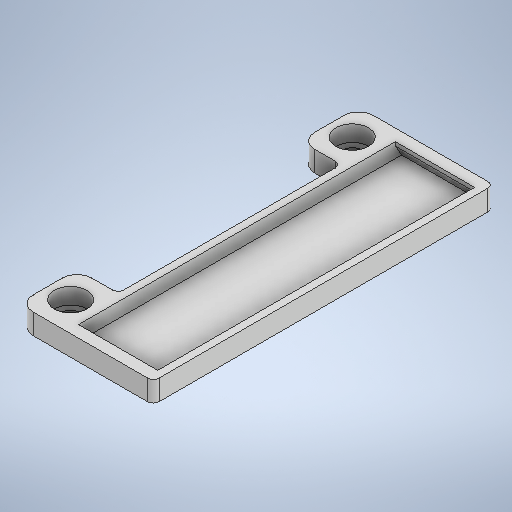
# Autodesk Inventor part: Bracket Clamp
Saved by Autodesk Inventor 2025 (Build 290162000, 162)
## iProperties
Created: 2025-03-11
Part Number: Bracket Clamp
Material: Generic
Document SubType Name: Modeling
Designer: Caleb Fangmeier
Density: 1 g/cm^3
Appearance: Default
Author: Caleb Fangmeier
Autodesk Inventor part; units mm, degrees
ref_plane "YZ Plane" through (0, 0, 0) normal (1, 0, 0) x (0, 1, 0)
ref_plane "XZ Plane" through (0, 0, 0) normal (0, 1, 0) x (-1, 0, 0)
ref_plane "XY Plane" through (0, 0, 0) normal (0, 0, 1) x (1, 0, 0)
sketch "Sketch1" plane through (0, 0, 0) normal (0, 1, 0) x (-1, 0, 0)
  line L0 (-16, 58) -> (16, 58)
  line L1 (16, 58) -> (16, -58)
  line L2 (16, -58) -> (-16, -58)
  line L3 (-16, -58) -> (-16, 58)
  line L4 (-16, 58) -> (16, -58) construction
  line L5 (16, 58) -> (-16, -58) construction
  point P0 (0, 0)
  dimension "d0" = 32
  dimension "d1" = 116
  constraints: 12 end point, 2 midpoint, 2 parallel, 1 horizontal, 1 perpendicular
  measures "d0" distance of L1.end L2.end
  measures "d1" distance of L0.end L1.end
extrude "Extrusion1" add sketch "Sketch1" along normal blind 7
sketch "Sketch3" plane through (16, 0, 58) normal (1, 0, 0) x (0, 0, -1)
  line L0 (0, 7) -> (116, 7) projected
  line L1 (4.75, 7) -> (1.8632, 2)
  line L2 (1.8632, 2) -> (114.1368, 2)
  line L3 (114.1368, 2) -> (111.25, 7)
  line L4 (0, 0) -> (0, 7) projected
  line L5 (116, 0) -> (116, 7) projected
  line L6 (4, 5.701) -> (4, 7)
  line L7 (116, 7) -> (0, 7) projected
  line L8 (112, 7) -> (112, 5.701)
  point P0 (58, 0)
  dimension "d4" = 60
  dimension "d6" = 60
  dimension "d7" = 5
  dimension "d8" = 106.5
  dimension "d9" = 116
  dimension "d10" = 4.75
  dimension "d17" = 4
  dimension "d18" = 4
  constraints: 10 end point, 6 point on line, 2 perpendicular, 1 horizontal
  measures "d4" angle of L2 L1
  measures "d6" angle of L2 L3
  measures "d7" distance between parallel lines of L0 L2
  measures "d8" distance of L1.start L3.end
  measures "d9" distance between parallel lines of L4 L5
  measures "d10" distance of L0.start L1.start
  measures "d17" distance between parallel lines of L4 L6
  measures "d18" distance between parallel lines of L8 L5
extrude "Extrusion2" cut sketch "Sketch3" against normal through all
sketch "Sketch4" plane through (0, 7, 0) normal (0, 1, 0) x (1, 0, 0)
  line L0 (-16, 58) -> (-16, -58) projected
  line L1 (-16, -58) -> (-13.5, -58)
  line L2 (-13.5, -58) -> (-13.5, 58)
  line L3 (-13.5, 58) -> (-16, 58)
  line L4 (-16, 58) -> (-16, -58)
  line L5 (16, -58) -> (16, 58) projected
  line L6 (16, -58) -> (13.5, -58)
  line L7 (13.5, -58) -> (13.5, 58)
  line L8 (13.5, 58) -> (16, 58)
  line L9 (16, 58) -> (16, -58)
  line L10 (16, 58) -> (-16, 58) projected
  point P0 (0, 0)
  dimension "d13" = 2.5
  dimension "d14" = 2.5
  constraints: 16 end point, 4 parallel, 2 horizontal, 2 perpendicular, 2 point on line
  measures "d13" distance between parallel lines of L5 L7
  measures "d14" distance between parallel lines of L0 L2
extrude "Extrusion3" add sketch "Sketch4" against normal up to surface (7 mm away)
sketch "Sketch5" plane through (0, 7, 0) normal (0, 1, 0) x (1, 0, 0)
  line L0 (-16, 58) -> (-16, -58) projected
  line L1 (-16, -58) -> (-25, -58)
  line L2 (-30, -53) -> (-30, -43)
  line L3 (-25, -38) -> (-16, -38)
  line L4 (-16, -38) -> (-16, -58)
  arc A0 (-30, -53) -> (-25, -58) centre (-25, -53) ccw
  arc A1 (-25, -38) -> (-30, -43) centre (-25, -43) ccw
  line L5 (-36.8459, 0) -> (21.1314, 0)
  line L6 (-16, 58) -> (-25, 58)
  line L7 (-30, 53) -> (-30, 43)
  line L8 (-25, 38) -> (-16, 38)
  line L9 (-16, 38) -> (-16, 58)
  arc A2 (-25, 58) -> (-30, 53) centre (-25, 53) ccw
  arc A3 (-30, 43) -> (-25, 38) centre (-25, 43) ccw
  point P0 (0, 0)
  point P1 (-30, -38)
  point P2 (-30, -58)
  point P3 (-22.2, -48)
  point P4 (-30, 38)
  point P5 (-30, 58)
  point P6 (-22.2, 48)
  dimension "d19" = 20
  dimension "d20" = 14
  dimension "d21" = 22.2
  dimension "d22" = 10
  dimension "d23" = 6.2
  dimension "d33" = 5
  constraints: 18 end point, 10 symmetric about line, 8 point on circle, 8 point on line, 4 centre point, 4 tangent, 2 horizontal, 2 parallel, 1 equal radius, 1 perpendicular, 2 other
  measures "d19" distance of point (-30, -58) point (-30, -38)
  measures "d20" distance of L0.end point (-30, -58)
  measures "d21" horizontal distance of point (-22.2, -48) point (0, 0)
  measures "d22" distance from line of point (-22.2, -48) L1
  measures "d23" distance from line of L0 point (-22.2, -48)
  measures "d33" radius of A0
extrude "Extrusion4" add sketch "Sketch5" against normal up to surface (7 mm away)
hole "Hole1" at (-22.2, 7, 48) at (-22.2, 7, -48) direction (0, -1, 0) diameter 6.756 depth 19.05 tip angle 118 counterbore diameter 11.113 counterbore depth 5.5 clearance for "Socket Head Cap Screw" size "1/4" standard "Ansi Unified Screw Threads"
fillet "Fillet1" radius 2 4 edges at (16, 3.5, -58) (16, 3.5, 58) (-16, 3.5, 38) (-16, 3.5, -38)
equation "\"d10\" = -0.5 * d8 + 0.5 * d9"
equation "\"d22\" = 0.5 * d19"
body "Solid1"
